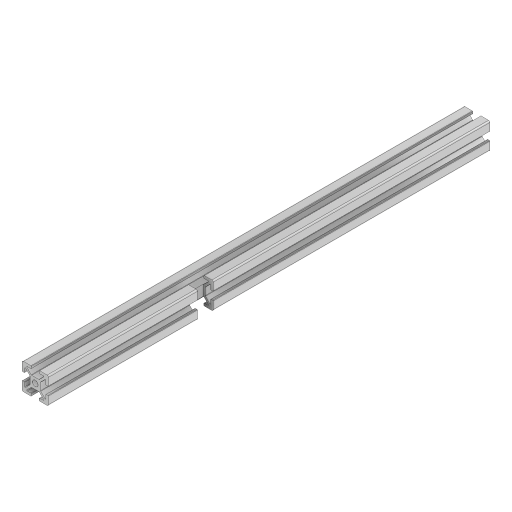
# Autodesk Inventor part: II Strebe waagrecht
Saved by Autodesk Inventor 2023 (Build 270158000, 158)
## iProperties
Created: 2022-09-26
Part Number: II Strebe waagrecht
Material: Aluminium 6061
Document SubType Name: Modeling
Designer: musati
Density: 2.7 g/cm^3
Appearance: Aluminum - Polished
Author: musati
Autodesk Inventor part; units mm, degrees
ref_plane "YZ Plane" through (0, 0, 0) normal (1, 0, 0) x (0, 1, 0)
ref_plane "XZ Plane" through (0, 0, 0) normal (0, 1, 0) x (-1, 0, 0)
ref_plane "XY Plane" through (0, 0, 0) normal (0, 0, 1) x (1, 0, 0)
sketch "Skizze1" plane through (0, 0, 0) normal (0, 0, 1) x (1, 0, 0)
  line L0 (-28.0083, 0) -> (28.0083, 0) projected
  line L1 (0, -28.0083) -> (0, 28.0083) projected
  line L2 (-20.0059, 0) -> (20.0059, 0)
  line L3 (0, -20.0059) -> (0, 20.0059)
  line L4 (-14.2899, 0) -> (14.2899, 0)
  line L5 (0, -14.2899) -> (0, 14.2899)
  line L6 (-10, -10) -> (10, 10) construction
  line L7 (10, -10) -> (-10, 10) construction
  line L8 (-8, -8) -> (8, 8) construction
  line L9 (8, -8) -> (-8, 8) construction
  line L10 (-2.7322, -4) -> (2.7322, -4)
  line L11 (4, -2.7322) -> (4, 2.7322)
  line L12 (2.7322, 4) -> (-2.7322, 4)
  line L13 (-4, 2.7322) -> (-4, -2.7322)
  line L14 (-4, -4) -> (4, 4) construction
  line L15 (4, -4) -> (-4, 4) construction
  arc A0 (-9, 10) -> (-10, 9) centre (-9, 9) ccw
  arc A1 (10, 9) -> (9, 10) centre (9, 9) ccw
  arc A2 (9, -10) -> (10, -9) centre (9, -9) ccw
  arc A3 (-10, -9) -> (-9, -10) centre (-9, -9) ccw
  line L16 (-3, 9.7) -> (-3, 8.3)
  line L17 (3, 9.7) -> (3, 8.3)
  line L18 (6.2151, 8) -> (3.3, 8)
  line L19 (-3.3, 8) -> (-6.2151, 8)
  line L20 (9, 10) -> (3.3, 10)
  line L21 (-3.3, 10) -> (-9, 10)
  line L22 (-9.7, -3) -> (-8.3, -3)
  line L23 (-9.7, 3) -> (-8.3, 3)
  line L24 (-8, 6.2151) -> (-8, 3.3)
  line L25 (-8, -3.3) -> (-8, -6.2151)
  line L26 (-10, 9) -> (-10, 3.3)
  line L27 (-10, -3.3) -> (-10, -9)
  line L28 (-3, -8.3) -> (-3, -9.7)
  line L29 (3, -8.3) -> (3, -9.7)
  line L30 (-9, -10) -> (-3.3, -10)
  line L31 (3.3, -10) -> (9, -10)
  line L32 (-6.2151, -8) -> (-3.3, -8)
  line L33 (3.3, -8) -> (6.2151, -8)
  line L34 (8.3, 3) -> (9.7, 3)
  line L35 (8.3, -3) -> (9.7, -3)
  line L36 (8, -6.2151) -> (8, -3.3)
  line L37 (8, 3.3) -> (8, 6.2151)
  line L38 (10, -9) -> (10, -3.3)
  line L39 (10, 3.3) -> (10, 9)
  arc A4 (-10, 3.3) -> (-9.7, 3) centre (-9.7, 3.3) ccw
  arc A5 (-8.3, 3) -> (-8, 3.3) centre (-8.3, 3.3) ccw
  arc A6 (-9.7, -3) -> (-10, -3.3) centre (-9.7, -3.3) ccw
  arc A7 (-8, -3.3) -> (-8.3, -3) centre (-8.3, -3.3) ccw
  arc A8 (-3.3, -10) -> (-3, -9.7) centre (-3.3, -9.7) ccw
  arc A9 (-3, -8.3) -> (-3.3, -8) centre (-3.3, -8.3) ccw
  arc A10 (3, -9.7) -> (3.3, -10) centre (3.3, -9.7) ccw
  arc A11 (3.3, -8) -> (3, -8.3) centre (3.3, -8.3) ccw
  arc A12 (8.3, -3) -> (8, -3.3) centre (8.3, -3.3) ccw
  arc A13 (10, -3.3) -> (9.7, -3) centre (9.7, -3.3) ccw
  arc A14 (8, 3.3) -> (8.3, 3) centre (8.3, 3.3) ccw
  arc A15 (9.7, 3) -> (10, 3.3) centre (9.7, 3.3) ccw
  arc A16 (3, 8.3) -> (3.3, 8) centre (3.3, 8.3) ccw
  arc A17 (3.3, 10) -> (3, 9.7) centre (3.3, 9.7) ccw
  arc A18 (-3.3, 8) -> (-3, 8.3) centre (-3.3, 8.3) ccw
  arc A19 (-3, 9.7) -> (-3.3, 10) centre (-3.3, 9.7) ccw
  line L40 (-7.4879, 6.4272) -> (-4.1464, 3.0858)
  line L41 (-6.4272, 7.4879) -> (-3.0858, 4.1464)
  line L42 (-6.4272, -7.4879) -> (-3.0858, -4.1464)
  line L43 (-7.4879, -6.4272) -> (-4.1464, -3.0858)
  arc A20 (-7.4879, 6.4272) -> (-8, 6.2151) centre (-7.7, 6.2151) ccw
  arc A21 (-6.2151, 8) -> (-6.4272, 7.4879) centre (-6.2151, 7.7) ccw
  arc A22 (-8, -6.2151) -> (-7.4879, -6.4272) centre (-7.7, -6.2151) ccw
  arc A23 (-6.4272, -7.4879) -> (-6.2151, -8) centre (-6.2151, -7.7) ccw
  line L44 (6.4272, -7.4879) -> (3.0858, -4.1464)
  line L45 (4.1464, -3.0858) -> (7.4879, -6.4272)
  arc A24 (6.2151, -8) -> (6.4272, -7.4879) centre (6.2151, -7.7) ccw
  arc A25 (7.4879, -6.4272) -> (8, -6.2151) centre (7.7, -6.2151) ccw
  line L46 (4.1464, 3.0858) -> (7.4879, 6.4272)
  line L47 (3.0858, 4.1464) -> (6.4272, 7.4879)
  arc A26 (6.4272, 7.4879) -> (6.2151, 8) centre (6.2151, 7.7) ccw
  arc A27 (8, 6.2151) -> (7.4879, 6.4272) centre (7.7, 6.2151) ccw
  arc A28 (-3.0858, 4.1464) -> (-2.7322, 4) centre (-2.7322, 4.5) ccw
  arc A29 (-4, 2.7322) -> (-4.1464, 3.0858) centre (-4.5, 2.7322) ccw
  arc A30 (2.7322, 4) -> (3.0858, 4.1464) centre (2.7322, 4.5) ccw
  arc A31 (4.1464, 3.0858) -> (4, 2.7322) centre (4.5, 2.7322) ccw
  arc A32 (-4.1464, -3.0858) -> (-4, -2.7322) centre (-4.5, -2.7322) ccw
  arc A33 (-2.7322, -4) -> (-3.0858, -4.1464) centre (-2.7322, -4.5) ccw
  arc A34 (3.0858, -4.1464) -> (2.7322, -4) centre (2.7322, -4.5) ccw
  arc A35 (4, -2.7322) -> (4.1464, -3.0858) centre (4.5, -2.7322) ccw
  circle A36 centre (0, 0) radius 2.1
  point P0 (-3, 9.1415)
  point P1 (3, 8.9014)
  point P2 (-8.9764, -3)
  point P3 (-9.1265, 3)
  point P4 (-3, -9.1251)
  point P5 (3, -9.1251)
  point P6 (9.1101, 3)
  point P7 (9.1101, -3)
  dimension "d0" = 20
  dimension "d1" = 20
  dimension "d2" = 16
  dimension "d3" = 16
  dimension "d4" = 8
  dimension "d5" = 8
  dimension "d6" = 1
  dimension "d7" = 6
  dimension "d8" = 6
  dimension "d9" = 6
  dimension "d10" = 6
  dimension "d11" = 0.3
  dimension "d12" = 1.5
  dimension "d13" = 1.5
  dimension "d14" = 0.3
  dimension "d15" = 1.5
  dimension "d16" = 0.3
  dimension "d17" = 1.5
  dimension "d18" = 0.3
  dimension "d19" = 0.5
  dimension "d20" = 4.2
  dimension "d21" = 45
  dimension "d22" = 10
  dimension "d23" = 10
  dimension "d24" = 4
  dimension "d25" = 4
  dimension "d26" = 10
  dimension "d27" = 8
  dimension "d28" = 4
  dimension "d29" = 4
  dimension "d30" = 10
  dimension "d31" = 9.1101
  dimension "d32" = 8
  dimension "d33" = 4
  dimension "d34" = 8.9014
  dimension "d35" = 9.1251
  dimension "d36" = 9.1415
  dimension "d37" = 8.9764
  dimension "d38" = 9.1265
  constraints: 92 end point, 90 tangent, 72 point on circle, 37 centre point, 30 equal radius, 23 parallel, 15 perpendicular, 8 point on line, 7 horizontal, 6 midpoint, 2 vertical, 1 coincident, 8 other
  measures "d0" distance of L7.end L6.end
  measures "d1" distance of L6.end L7.start
  measures "d2" distance of L9.end L8.end
  measures "d3" distance of L8.end L9.start
  measures "d4" distance of L15.end L14.end
  measures "d5" distance of L14.end L15.start
  measures "d6" radius of A0
  measures "d7" horizontal distance of point (3, 8.901) point (-3, 9.142)
  measures "d8" vertical distance of point (-8.976, -3) point (-9.127, 3)
  measures "d9" distance of point (3, -9.125) point (-3, -9.125)
  measures "d10" distance of point (9.11, -3) point (9.11, 3)
  measures "d11" radius of A4
  measures "d12" distance between parallel lines of L41 L40
  measures "d13" distance between parallel lines of L43 L42
  measures "d14" radius of A20
  measures "d15" distance between parallel lines of L44 L45
  measures "d16" radius of A24
  measures "d17" distance between parallel lines of L47 L46
  measures "d18" radius of A26
  measures "d19" radius of A28
  measures "d20" diameter of A36
  measures "d21" angle of L45 L5
  measures "d22" distance between parallel lines of L39 L5
  measures "d23" distance between parallel lines of L20 L4
  measures "d24" distance between parallel lines of L10 L4
  measures "d25" distance between parallel lines of L13 L5
  measures "d26" distance between parallel lines of L27 L5
  measures "d27" distance between parallel lines of L32 L4
  measures "d28" distance between parallel lines of L11 L5
  measures "d29" distance between parallel lines of L12 L4
  measures "d30" distance from line of L6.end L5
  measures "d31" distance from line of point (9.11, 3) L5
  measures "d32" distance from line of L8.end L5
  measures "d33" distance from line of L14.end L5
  measures "d34" distance from line of point (3, 8.901) L4
  measures "d35" distance from line of point (3, -9.125) L4
  measures "d36" distance from line of point (-3, 9.142) L4
  measures "d37" distance from line of point (-8.976, -3) L5
  measures "d38" distance from line of point (-9.127, 3) L5
extrude "Extrusion1" add sketch "Skizze1" against normal blind 335 contours L13 A29 L40 A20 L24 A5 L23 A4 L26 A0 L21 A19 L16 A18 L19 A21 L41 A28 L12 L1 A36 L0 | L0 A36 L1 L10 A33 L42 A23 L32 A9 L28 A8 L30 A3 L27 A6 L22 A7 L25 A22 L43 A32 L13 | L1 L12 A30 L47 A26 L18 A16 L17 A17 L20 A1 L39 A15 L34 A14 L37 A27 L46 A31 L11 L0 A36 | A36 L0 L11 A35 L45 A25 L36 A12 L35 A13 L38 A2 L31 A10 L29 A11 L33 A24 L44 A34 L10 L1
sketch "Skizze2" plane through (9, 10, 0) normal (0, 1, 0) x (1, 0, 0)
  line L0 (0, 0) -> (-5.7, 0) projected
  line L1 (0, 0) -> (0, 335) projected
  line L2 (-5.7, 335) -> (0, 335) projected
  line L3 (-5.7, 0) -> (-5.7, 335) projected
  line L4 (-12.3, 0) -> (-18, 0) projected
  line L5 (-12.3, 0) -> (-12.3, 335) projected
  line L6 (-18, 335) -> (-12.3, 335) projected
  line L7 (-18, 0) -> (-18, 335) projected
  line L8 (-6.2678, 0) -> (-6.2678, 335) projected
  line L9 (-23, 0) -> (5, 0) projected
  line L10 (-9, 402) -> (-9, -67) projected
  line L11 (1, 0) -> (1, 335) projected
  line L12 (1, 113) -> (-6.5, 113)
  line L13 (-6.5, 113) -> (-6.5, 125)
  line L14 (-6.5, 125) -> (1, 125)
  line L15 (1, 125) -> (1, 113)
  point P0 (-9, 0)
  point P1 (1, 125)
  dimension "d41" = 7.5
  dimension "d42" = 12
  dimension "d43" = 210
  constraints: 8 end point, 2 parallel, 1 horizontal, 1 perpendicular, 1 point on line, 1 other
  measures "d41" distance of L13.end L14.end
  measures "d42" distance of L12.end L13.end
  measures "d43" distance between parallel lines of L14 L2
extrude "Extrusion2" cut sketch "Skizze2" against normal blind 335 contours L12 L3 L14 L1 | L1 L14 L11 L12 | L12 L8 L14 L3 | L12 L13 L14 L8
